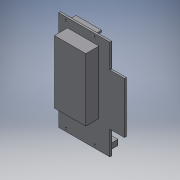
# Autodesk Inventor part: pcb
Saved by Autodesk Inventor 2017 (Build 210142000, 142)
## iProperties
Created: 2017-06-09
Part Number: pcb
Material: Ogólny
Document SubType Name: Modeling
Designer: Speed King
Density: 1 g/cm^3
Appearance: Domyślna
Author: Speed King
Autodesk Inventor part; units mm, degrees
ref_plane "YZ Plane" through (0, 0, 0) normal (1, 0, 0) x (0, 1, 0)
ref_plane "XZ Plane" through (0, 0, 0) normal (0, 1, 0) x (-1, 0, 0)
ref_plane "XY Plane" through (0, 0, 0) normal (0, 0, 1) x (1, 0, 0)
sketch "Szkic1" plane through (0, 0, 0) normal (0, 1, 0) x (-1, 0, 0)
  line L0 (-35, -68) -> (35, -68)
  line L1 (35, -68) -> (35, 68)
  line L2 (35, 68) -> (-35, 68)
  line L3 (-35, 68) -> (-35, -68)
  line L4 (-35, -68) -> (35, 68) construction
  line L5 (35, -68) -> (-35, 68) construction
  point P0 (0, 0)
  dimension "d0" = 70
  dimension "d1" = 136
  constraints: 12 end point, 2 midpoint, 2 parallel, 1 horizontal, 1 perpendicular
  measures "d0" distance of L2.end L1.end
  measures "d1" distance of L1.end L0.end
extrude "Wyciągnięcie proste1" add sketch "Szkic1" along normal blind 2.5
sketch "Szkic2" plane through (0, 2.5, 0) normal (0, 1, 0) x (1, 0, 0)
  line L0 (-52.8, 0) -> (71.8, 0) projected
  line L1 (35, -68) -> (35, 68) projected
  line L2 (55, -35) -> (35, -35)
  line L3 (35, -35) -> (35, 35)
  line L4 (35, 35) -> (55, 35)
  line L5 (55, 35) -> (55, -35)
  line L6 (55, -35) -> (35, 35) construction
  line L7 (35, -35) -> (55, 35) construction
  point P0 (0, 0)
  point P1 (45, 0)
  dimension "d4" = 20
  dimension "d5" = 70
  constraints: 12 end point, 2 midpoint, 2 parallel, 2 point on line, 1 horizontal, 1 perpendicular
  measures "d4" distance between parallel lines of L1 L5
  measures "d5" distance between parallel lines of L2 L4
extrude "Wyciągnięcie proste2" add sketch "Szkic2" against normal up to surface (2.5 mm away)
sketch "Szkic3" plane through (0, 2.5, 0) normal (0, 1, 0) x (1, 0, 0)
  circle A0 centre (-25, 64) radius 1.3
  line L0 (35, 68) -> (-35, 68) projected
  line L1 (-35, -68) -> (35, -68) projected
  line L2 (-35, 68) -> (-35, -68) projected
  circle A1 centre (14.5, 64) radius 1.3
  circle A2 centre (-25, -64) radius 1.3
  circle A3 centre (14.5, -64) radius 1.3
  point P0 (0, 0)
  dimension "d8" = 2.6
  dimension "d9" = 4
  dimension "d10" = 136
  dimension "d13" = 39.5
  dimension "d16" = 128
  dimension "d19" = 10
  constraints: 4 centre point, 1 horizontal, 1 vertical, 6 other
  measures "d8" diameter of A0
  measures "d9" distance from line of A0.centre L0
  measures "d10" distance between parallel lines of L1 L0
  measures "d13" distance of A0.centre A1.centre
  measures "d16" distance of A0.centre A2.centre
  measures "d19" distance from line of L2 A0.centre
extrude "Wyciągnięcie proste3" cut sketch "Szkic3" against normal up to next
sketch "Szkic4" plane through (0, 2.5, 0) normal (0, 1, 0) x (1, 0, 0)
  line L0 (-23, -65) -> (12, -65)
  line L1 (12, -65) -> (12, -62.5)
  line L2 (12, -62.5) -> (-23, -62.5)
  line L3 (-23, -62.5) -> (-23, -65)
  line L4 (-23, -65) -> (12, -62.5) construction
  line L5 (12, -65) -> (-23, -62.5) construction
  line L6 (-35, -68) -> (35, -68) projected
  line L7 (-35, 68) -> (-35, -68) projected
  point P0 (0, 0)
  point P1 (-5.5, -63.75)
  dimension "d22" = 35
  dimension "d23" = 2.5
  dimension "d24" = 3
  dimension "d25" = 12
  constraints: 12 end point, 2 midpoint, 2 parallel, 1 horizontal, 1 perpendicular
  measures "d22" distance of L2.end L1.end
  measures "d23" distance of L1.end L0.end
  measures "d24" distance between parallel lines of L6 L0
  measures "d25" distance between parallel lines of L7 L3
extrude "Wyciągnięcie proste4" add sketch "Szkic4" along normal blind 9
sketch "Szkic5" plane through (0, 2.5, 0) normal (0, 1, 0) x (1, 0, 0)
  line L0 (-29.5, -54) -> (-23.5, -54)
  line L1 (-23.5, -54) -> (-23.5, 27)
  line L2 (-23.5, 27) -> (-29.5, 27)
  line L3 (-29.5, 27) -> (-29.5, -54)
  line L4 (-29.5, -54) -> (-23.5, 27) construction
  line L5 (-23.5, -54) -> (-29.5, 27) construction
  line L6 (-35, -68) -> (35, -68) projected
  line L7 (-35, 68) -> (-35, -68) projected
  line L8 (17, -54) -> (23, -54)
  line L9 (23, -54) -> (23, 27)
  line L10 (23, 27) -> (17, 27)
  line L11 (17, 27) -> (17, -54)
  line L12 (17, -54) -> (23, 27) construction
  line L13 (23, -54) -> (17, 27) construction
  line L14 (35, -68) -> (35, -35) projected
  point P0 (0, 0)
  point P1 (-26.5, -13.5)
  point P2 (20, -13.5)
  dimension "d28" = 6
  dimension "d29" = 81
  dimension "d30" = 14
  dimension "d31" = 5.5
  dimension "d32" = 6
  dimension "d33" = 81
  dimension "d34" = 14
  dimension "d35" = 12
  constraints: 24 end point, 4 midpoint, 4 parallel, 2 horizontal, 2 perpendicular
  measures "d28" distance of L2.end L1.end
  measures "d29" distance of L1.end L0.end
  measures "d30" distance between parallel lines of L6 L0
  measures "d31" distance between parallel lines of L7 L3
  measures "d32" distance of L10.end L9.end
  measures "d33" distance of L9.end L8.end
  measures "d34" distance between parallel lines of L6 L8
  measures "d35" distance between parallel lines of L14 L9
extrude "Wyciągnięcie proste5" add sketch "Szkic5" along normal blind 9
sketch "Szkic6" plane through (0, 2.5, 0) normal (0, 1, 0) x (1, 0, 0)
  line L0 (32.5, 55) -> (17.5, 55)
  line L1 (17.5, 55) -> (17.5, 62.5)
  line L2 (17.5, 62.5) -> (32.5, 62.5)
  line L3 (32.5, 62.5) -> (32.5, 55)
  line L4 (32.5, 55) -> (17.5, 62.5) construction
  line L5 (17.5, 55) -> (32.5, 62.5) construction
  line L6 (11, 62.5) -> (1, 62.5)
  line L7 (1, 62.5) -> (1, 55)
  line L8 (1, 55) -> (11, 55)
  line L9 (11, 55) -> (11, 62.5)
  line L10 (11, 62.5) -> (1, 55) construction
  line L11 (1, 62.5) -> (11, 55) construction
  line L12 (35, 35) -> (35, 68) projected
  line L13 (35, 68) -> (-35, 68) projected
  point P0 (0, 0)
  point P1 (25, 58.75)
  point P2 (6, 58.75)
  dimension "d38" = 15
  dimension "d39" = 7.5
  dimension "d40" = 10
  dimension "d41" = 7.5
  dimension "d42" = 6.5
  dimension "d43" = 2.5
  dimension "d44" = 5.5
  dimension "d45" = 5.5
  constraints: 24 end point, 4 midpoint, 4 parallel, 2 horizontal, 2 perpendicular
  measures "d38" distance of L1.end L2.end
  measures "d39" distance of L0.end L1.end
  measures "d40" distance of L8.end L7.end
  measures "d41" distance of L7.end L6.end
  measures "d42" distance between parallel lines of L9 L1
  measures "d43" distance between parallel lines of L3 L12
  measures "d44" distance between parallel lines of L2 L13
  measures "d45" distance between parallel lines of L6 L13
extrude "Wyciągnięcie proste6" add sketch "Szkic6" along normal blind 11
sketch "Szkic7" plane through (0, 2.5, 0) normal (0, 1, 0) x (1, 0, 0)
  line L0 (-0.5, 65.5) -> (-14.5, 65.5)
  line L1 (-14.5, 65.5) -> (-14.5, 63)
  line L2 (-14.5, 63) -> (-0.5, 63)
  line L3 (-0.5, 63) -> (-0.5, 65.5)
  line L4 (-0.5, 65.5) -> (-14.5, 63) construction
  line L5 (-14.5, 65.5) -> (-0.5, 63) construction
  line L6 (35, 68) -> (-35, 68) projected
  line L7 (-35, 68) -> (-35, -68) projected
  point P0 (0, 0)
  point P1 (-7.5, 64.25)
  dimension "d48" = 14
  dimension "d49" = 2.5
  dimension "d50" = 2.5
  dimension "d51" = 20.5
  constraints: 12 end point, 2 midpoint, 2 parallel, 1 horizontal, 1 perpendicular
  measures "d48" distance of L2.end L1.end
  measures "d49" distance of L1.end L0.end
  measures "d50" distance between parallel lines of L0 L6
  measures "d51" distance between parallel lines of L7 L1
extrude "Wyciągnięcie proste7" add sketch "Szkic7" along normal blind 9
sketch "Szkic8" plane through (0, 0, 0) normal (0, -1, 0) x (1, 0, 0)
  line L0 (20, 56) -> (-23, 56)
  line L1 (-23, 56) -> (-23, -30)
  line L2 (-23, -30) -> (20, -30)
  line L3 (20, -30) -> (20, 56)
  line L4 (20, 56) -> (-23, -30) construction
  line L5 (-23, 56) -> (20, -30) construction
  line L6 (-35, 68) -> (35, 68) projected
  line L7 (-35, -68) -> (-35, 68) projected
  point P0 (0, 0)
  point P1 (-1.5, 13)
  dimension "d54" = 43
  dimension "d55" = 86
  dimension "d56" = 12
  dimension "d57" = 12
  constraints: 12 end point, 2 midpoint, 2 parallel, 1 horizontal, 1 perpendicular
  measures "d54" distance of L2.end L1.end
  measures "d55" distance of L1.end L0.end
  measures "d56" distance between parallel lines of L6 L0
  measures "d57" distance between parallel lines of L1 L7
extrude "Wyciągnięcie proste8" add sketch "Szkic8" along normal blind 18
equation "\"d16\" = d10 - 2 * d9"
equation "\"d45\" = d44"
